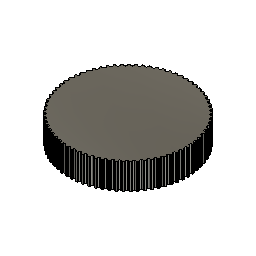
gear_73z (Autodesk Fusion 360 design; units mm, degrees)
Autodesk Fusion 360 part; units mm, degrees
sketch "Sketch1" plane through (0, 0, 0) normal (0, 0, 1) x (1, 0, 0) in component "gt2 pulley"
  circle A0 centre (0, 0) radius 23.2366 construction
  circle A1 centre (0, 0) radius 22.2326 construction
  line L0 (0, 0) -> (0, 23.2366) construction
  line L1 (0, 0) -> (0.9997, 23.2151) construction
  line L2 (0, 0) -> (1.4053, 23.1941) construction
  circle A2 centre (0, 0) radius 22.9826 construction
  arc A3 (0.3945, 22.8456) -> (0.4696, 22.5495) centre (1.3899, 22.9406) ccw
  circle A4 centre (0, 0) radius 22.8326 construction
  arc A5 (0.2467, 22.9813) -> (0, 22.9826) centre (0, 0) ccw
  arc A6 (0.3945, 22.8456) -> (0.2467, 22.9813) centre (0.2451, 22.8313) ccw
  arc A7 (0.4696, 22.5495) -> (0.9565, 22.212) centre (0.9804, 22.7665) ccw
  arc A8 (0, 22.9826) -> (-0.2467, 22.9813) centre (0, 0) ccw
  arc A9 (-0.2467, 22.9813) -> (-0.3945, 22.8456) centre (-0.2451, 22.8313) ccw
  arc A10 (-0.4696, 22.5495) -> (-0.3945, 22.8456) centre (-1.3899, 22.9406) ccw
  arc A11 (-0.9565, 22.212) -> (-0.4696, 22.5495) centre (-0.9804, 22.7665) ccw
  arc A12 (0.9565, 22.212) -> (-0.9565, 22.212) centre (0, 0) ccw
  point P0 (1.3899, 22.9406)
  point P1 (0, 22.9826)
  dimension "d18" = 46.4732
  dimension "d19" = 2.466
  dimension "d22" = 1.004
  dimension "d24" = 0.75
  dimension "d26" = 1
  dimension "d27" = 0.15
  dimension "d28" = 0.15
  dimension "d47" = 0.555
  dimension "d52" = 3.812
  constraint coincident A0.centre A1.centre
  constraint coincident A0 L0.end
  constraint vertical L0
  constraint coincident A0 L1.end
  constraint coincident A0 L2.end
  constraint concentric A1 A2
  constraint coincident A1 A7.end
  constraint coincident L1 A7.end
  constraint coincident A2 P0
  constraint coincident L2 P0
  constraint coincident P0 A3.centre
  constraint coincident A2 P1
  constraint coincident L0 P1
  constraint concentric A2 A4
  constraint coincident P1 A5.end
  constraint coincident A4 A6.centre
  constraint coincident A3.start A6.start
  constraint tangent A3 A6
  constraint tangent A3 A7
  constraint symmetric L0 A7.end A11.start
  constraint symmetric L0 A3.start A9.end
  constraint symmetric L0 A3.end A10.start
  constraint symmetric L0 A3 A10
  constraint symmetric L0 A5.start A8.end
  constraint symmetric L0 P1 A5.end
  constraint symmetric L0 A5 A8
  constraint symmetric L0 A6 A9
  constraint symmetric L0 A7 A11
  constraint coincident A1 A11.start
  constraint tangent A1 A7
  constraint coincident L1 A7.centre
  measures "d18" diameter of A0
  measures "d19" angle of L0 L1
  measures "d22" distance of A0 A1
  measures "d24" distance of A1 A2
  measures "d26" radius of A3
  measures "d27" distance of A2 A4
  measures "d28" radius of A6
  measures "d47" radius of A7
extrude "Extrude1" add sketch "Sketch1" along normal blind 10 makes body 1
pattern_circular "C-Pattern1" count 73 over 360 about axis through (0, 0, 1.75) along (0, 0, 1) of bodies 1 makes body 2 at (-1.1689, 22.2019, 3.3333) makes body 3 at (-3.913, 21.8856, 6.6667) makes body 4 at (-4.9546, 21.6735, 3.3333) makes body 5 at (-7.4039, 20.9636, 6.6667) makes body 6 at (-8.5939, 20.5045, 3.3333) makes body 7 at (-10.3248, 19.6898, 3.3333) makes body 8 at (-11.9792, 18.7294, 6.6667) makes body 9 at (-14.2093, 17.0993, 6.6667) makes body 10 at (-15.6266, 15.8145, 6.6667) makes body 11 at (-17.3347, 13.9211, 6.6667) makes body 12 at (-18.1046, 12.9041, 6.6667) makes body 13 at (-19.1468, 11.2999, 6.6667) makes body 14 at (-20.0473, 9.6121, 6.6667) makes body 15 at (-20.7994, 7.8532, 6.6667) makes body 16 at (-21.151, 6.85, 3.3333) makes body 17 at (-21.8372, 4.1743, 6.6667) makes body 18 at (-22.1152, 2.2816, 6.6667) makes body 19 at (-22.2295, 0.3721, 6.6667) makes body 20 at (-22.1792, -1.5403, 6.6667) makes body 21 at (-22.0802, -2.5986, 3.3333) makes body 22 at (-21.7751, -4.4872, 3.3333) makes body 23 at (-21.3088, -6.3424, 6.6667) makes body 24 at (-20.0931, -9.5162, 6.6667) makes body 25 at (-19.3069, -11.0241, 6.6667) makes body 26 at (-18.5263, -12.2909, 6.6667) makes body 27 at (-17.4011, -13.8381, 6.6667) makes body 28 at (-15.702, -15.7396, 6.6667) makes body 29 at (-14.2909, -17.0312, 6.6667) makes body 30 at (-13.9625, -17.3014, 3.3333) makes body 31 at (-12.4235, -18.4376, 6.6667) makes body 32 at (-10.7925, -19.4374, 3.3333) makes body 33 at (-9.0817, -20.2932, 3.3333) makes body 34 at (-7.3035, -20.9988, 3.3333) makes body 35 at (-5.4713, -21.5489, 3.3333) makes body 36 at (-2.9678, -22.0336, 6.6667) makes body 37 at (-0.8503, -22.2164, 6.6667) makes body 38 at (1.0627, -22.2072, 6.6667) makes body 39 at (2.757, -22.061, 6.6667) makes body 40 at (4.0176, -21.8666, 3.3333) makes body 41 at (6.6982, -21.1996, 6.6667) makes body 42 at (8.4958, -20.5453, 6.6667) makes body 43 at (9.4681, -20.1158, 3.3333) makes body 44 at (11.1623, -19.2274, 6.6667) makes body 45 at (13.9625, -17.3014, 6.6667) makes body 46 at (14.9317, -16.4722, 6.6667) makes body 47 at (15.702, -15.7396, 3.3333) makes body 48 at (17.5326, -13.671, 6.6667) makes body 49 at (18.166, -12.8173, 3.3333) makes body 50 at (19.2006, -11.2083, 3.3333) makes body 51 at (20.6846, -8.1508, 6.6667) makes body 52 at (20.8368, -7.7537, 6.6667) makes body 53 at (21.4262, -5.9337, 3.3333) makes body 54 at (22.0802, -2.5986, 6.6667) makes body 55 at (22.1929, -1.3281, 6.6667) makes body 56 at (22.231, -0.2658, 3.3333) makes body 57 at (22.1716, 1.6463, 3.3333) makes body 58 at (21.7963, 4.383, 6.6667) makes body 59 at (21.3388, 6.2405, 6.6667) makes body 60 at (21.0162, 7.2533, 3.3333) makes body 61 at (20.3148, 9.0331, 3.3333) makes body 62 at (18.7007, 12.0239, 6.6667) makes body 63 at (17.5978, 13.587, 6.6667) makes body 64 at (16.3646, 15.0495, 6.6667) makes body 65 at (15.4746, 15.9632, 6.6667) makes body 66 at (14.0451, 17.2344, 6.6667) makes body 67 at (13.2052, 17.8861, 6.6667) makes body 68 at (10.8854, 19.3855, 6.6667) makes body 69 at (9.9463, 19.8837, 3.3333) makes body 70 at (7.604, 20.8918, 6.6667) makes body 71 at (4.9546, 21.6735, 6.6667) makes body 72 at (4.5392, 21.7643, 3.3333) makes body 73 at (2.6514, 22.074, 3.3333)
sketch "Sketch2" plane through (0, 0, 10) normal (0, 0, 1) x (-1, 0, 0)
  arc A0 (-14.8214, -17.3897) -> (-14.7935, -17.5884) centre (-14.697, -17.4736) ccw
  arc A1 (-14.7935, -17.5884) -> (-14.4126, -17.9019) centre (0, 0) ccw
  arc A2 (-14.4126, -17.9019) -> (-14.2122, -17.891) centre (-14.3185, -17.7851) ccw
  arc A3 (-13.9661, -17.7101) -> (-14.2122, -17.891) centre (-13.5039, -18.5969) ccw
  arc A4 (-13.3757, -17.759) -> (-13.9661, -17.7101) centre (-13.7096, -18.2023) ccw
  arc A5 (-14.8528, -16.5434) -> (-13.3757, -17.759) centre (0, 0) ccw
  arc A6 (-14.6913, -17.1133) -> (-14.8528, -16.5434) centre (-15.2236, -16.9564) ccw
  arc A7 (-14.8214, -17.3897) -> (-14.6913, -17.1133) centre (-15.6504, -16.8305) ccw
  circle A8 centre (0, 0) radius 22.2326
  constraint concentric A1 A8
extrude "Extrude2" add sketch "Sketch2" against normal blind 10 contours A5 A8 bodies 1 2 3 4 5 6 7 8 9 10 11 12 13 14 15 16 17 18 19 20 21 22 23 24 25 26 27 28 29 30 31 32 33 34 35 36 37 38 39 40 41 42 43 44 45 46 47 48 49 50 51 52 53 54 55 56 57 58 59 60 61 62 63 64 65 66 67 68 69 70 71 72 73
extrude "Extrude4" [suppressed] in component "gt2 pulley"
pattern_circular "C-Pattern7" [suppressed] in component "gt2 pulley"
extrude "Extrude3" [suppressed] in component "gt2 pulley"
pattern_circular "C-Pattern6" [suppressed] in component "gt2 pulley"
extrude "Extrude2'" [suppressed] in component "gt2 pulley"
pattern_circular "C-Pattern5" [suppressed] in component "gt2 pulley"
extrude "Extrude1'" [suppressed] in component "gt2 pulley"
pattern_circular "C-Pattern4" [suppressed] in component "gt2 pulley"
pattern_circular "C-Pattern3" [suppressed] in component "gt2 pulley"
pattern_circular "C-Pattern2" [suppressed] in component "gt2 pulley"
pattern_circular "C-Pattern1'" [suppressed] in component "gt2 pulley"
copy_body "Body->Comp1" [suppressed] in component "Component"
copy_body "Body->Comp2" [suppressed] in component "Component'"
copy_body "Body->Comp3" [suppressed] in component "Component''"
copy_body "Body->Comp4" [suppressed] in component "Component'''"
copy_body "Body->Comp5" [suppressed] in component "Component''''"
copy_body "Body->Comp6" [suppressed] in component "Component'''''"
copy_body "Body->Comp7" [suppressed] in component "Component''''''"
copy_body "Body->Comp8" [suppressed] in component "Component'''''''"
copy_body "Body->Comp9" [suppressed] in component "Component''''''''"
copy_body "Body->Comp10" [suppressed] in component "Component'''''''''"
copy_body "Body->Comp11" [suppressed] in component "Component''''''''''"
copy_body "Body->Comp12" [suppressed] in component "Component'''''''''''"
copy_body "Body->Comp13" [suppressed] in component "Component''''''''''''"
copy_body "Body->Comp14" [suppressed] in component "Component'''''''''''''"
copy_body "Body->Comp15" [suppressed] in component "Component''''''''''''''"
copy_body "Body->Comp16" [suppressed] in component "Component'''''''''''''''"
copy_body "Body->Comp17" [suppressed] in component "Component''''''''''''''''"
copy_body "Body->Comp18" [suppressed] in component "Component'''''''''''''''''"
copy_body "Body->Comp19" [suppressed] in component "Component''''''''''''''''''"
copy_body "Body->Comp20" [suppressed] in component "Component'''''''''''''''''''"
component "gt2 pulley" placed x (1, 0, 0) y (0, 1, 0) z (0, 0, 1) at (0, 0, 0)
equation "NumTeeth = 73" comment "min 20"
equation "ToothPitch = 2 mm"
equation "PullyDia = NumTeeth * ToothPitch / PI"
equation "ToothAng = ( ( 360 / NumTeeth ) * 1 deg )"
equation "TransOffsetAngle = ToothAng * 0.2"
equation "Sholulder_Radius = 0.15 mm"
equation "Root_Radius = 0.555 mm"
equation "TransRadius = 1 mm"
equation "ToolHeight = 0.75 mm"
equation "PLD = 0.254 mm"
equation "d18 = PullyDia"
equation "d19 = ToothAng / 2"
equation "d22 = PLD + ToolHeight"
equation "d24 = ToolHeight"
equation "d26 = TransRadius"
equation "d27 = Sholulder_Radius"
equation "d31 = NumTeeth"
equation "d33 = NumTeeth"
equation "d35 = NumTeeth"
equation "d37 = NumTeeth"
equation "d41 = NumTeeth"
equation "d45 = NumTeeth"
equation "d47 = Root_Radius"
equation "d50 = NumTeeth"
